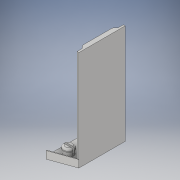
# Autodesk Inventor part: SOPORTE
Saved by Autodesk Inventor 2019 (Build 230136000, 136)
## iProperties
Created: 2020-12-03
Part Number: SOPORTE
Material: Generic
Document SubType Name: Modeling
Designer: mihai
Density: 1 g/cm^3
Appearance: Default
Author: mihai
Autodesk Inventor part; units mm, degrees
ref_plane "YZ Plane" through (0, 0, 0) normal (1, 0, 0) x (0, 1, 0)
ref_plane "XZ Plane" through (0, 0, 0) normal (0, 1, 0) x (-1, 0, 0)
ref_plane "XY Plane" through (0, 0, 0) normal (0, 0, 1) x (1, 0, 0)
sketch "Sketch1" plane through (0, 0, 0) normal (0, 1, 0) x (-1, 0, 0)
  line L0 (0, 0) -> (0, -30)
  circle A0 centre (0, 5) radius 5
  circle A1 centre (0, -35) radius 5
  line L1 (-5, 5) -> (-14, 5) construction
  line L2 (0, 10) -> (0, 15) construction
  line L3 (0, 10) -> (-14, 10) construction
  line L4 (5, 5) -> (10, 5) construction
  line L5 (-14, 5) -> (-11.1, 5) construction
  line L6 (0, 0) -> (-14, 0) construction
  line L7 (-11.1, 0) -> (-11.1, 1) construction
  line L8 (5, -35) -> (10, -35) construction
  line L9 (0, -40) -> (0, -45) construction
  line L10 (-5, -35) -> (-14, -35) construction
  line L11 (0, -40) -> (-14, -40) construction
  line L12 (0, -30) -> (-14, -30) construction
  line L13 (-11.1, -30) -> (-11.1, -31) construction
  line L14 (-14, 10) -> (0, 15)
  line L15 (0, 15) -> (10, 18.5714)
  line L16 (-14, -40) -> (0, -45)
  line L17 (0, -45) -> (10, -48.5714)
  line L18 (10, -48.5714) -> (10, 18.5714)
  line L19 (-14, 10) -> (-14, 5)
  line L20 (-11.1, 1) -> (-11.1, -31)
  line L21 (-14, -40) -> (-14, -35)
  line L22 (-14, 10) -> (-14, 3.9) construction
  line L23 (-14, -40) -> (-14, -33.9) construction
  line L24 (-11.1, 1) -> (-14, 4.45)
  line L25 (-11.1, -31) -> (-14, -34.45)
  line L26 (-14, 4.45) -> (-14, 5)
  line L27 (-14, -34.45) -> (-14, -35)
  dimension "d0" = 30
  dimension "d3" = 9
  dimension "d4" = 5
  dimension "d5" = 5
  dimension "d6" = 2.9
  dimension "d7" = 1
  dimension "d8" = 5
  dimension "d9" = 1
  dimension "d10" = 6.1
  dimension "d11" = 6.1
  constraints: 56 end point, 9 point on circle, 8 horizontal, 7 point on line, 5 vertical, 2 centre point, 2 collinear, 2 parallel, 2 tangent, 1 perpendicular
  measures "d0" distance of L0.start L0.end
  measures "d3" distance of L1.start L1.end
  measures "d4" distance of L2.start L2.end
  measures "d5" distance of L4.start L4.end
  measures "d6" distance of L1.end L5.end
  measures "d7" distance of L7.start L7.end
  measures "d8" distance of L9.start L9.end
  measures "d9" distance of L13.start L13.end
  measures "d10" distance of L3.end L22.end
  measures "d11" distance of L11.end L23.end
extrude "Extrusion3" add sketch "Sketch1" along normal blind 3
sketch "Sketch4" plane through (0, 3, 0) normal (0, 1, 0) x (1, 0, 0)
  circle A0 centre (0, 35) radius 5 projected
  circle A1 centre (0, -5) radius 5 projected
  point P0 (0, 0)
  constraints: 1 vertical alignment
sketch "Sketch5" plane through (0, 3, 0) normal (0, 1, 0) x (1, 0, 0)
  point P0 (0, 0)
extrude "Extrusion4" add sketch "Sketch4" along normal blind 5
sketch "Sketch6" plane through (0, 8, 5) normal (0, 1, 0) x (1, 0, 0)
  circle A0 centre (0, 0) radius 5.5
  circle A1 centre (0, 40) radius 5 projected
  circle A2 centre (0, 40) radius 5.5
  point P0 (0, 5)
  dimension "d20" = 11
  dimension "d21" = 11
  constraints: 2 centre point, 1 coincident
  measures "d20" diameter of A0
  measures "d21" diameter of A2
extrude "Extrusion5" add sketch "Sketch6" along normal blind 3 contours A0 | A1 | A2
fillet "Fillet1" radius 2 2 edges at (-5.5, 11, 5) (-5.5, 11, -35)
sketch "Sketch7" plane through (0, 11, 5) normal (0, 1, 0) x (1, 0, 0)
  circle A0 centre (0, 0) radius 3.5 projected
  circle A1 centre (0, 40) radius 3.5 projected
  circle A2 centre (0, 0) radius 5.5 projected
  line L0 (-5.5, 0) -> (-5.5, 1)
  line L1 (-5.5, 1) -> (5.5, 1)
  line L2 (5.5, 1) -> (5.5, -1)
  line L3 (5.5, -1) -> (-5.5, -1)
  line L4 (-5.5, -1) -> (-5.5, 0)
  line L5 (-5.5, 40) -> (-5.5, 41)
  line L6 (-5.5, 41) -> (5.5, 41)
  line L7 (5.5, 41) -> (5.5, 39)
  line L8 (5.5, 39) -> (-5.5, 39.0974)
  line L9 (-5.5, 39.0974) -> (-5.5, 40)
  circle A3 centre (0, 40) radius 5.5 projected
  point P0 (0, 5)
  dimension "d25" = 1
  dimension "d26" = 2
  dimension "d27" = 1
  dimension "d28" = 2
  constraints: 20 end point, 6 point on line, 5 perpendicular, 4 vertical, 2 horizontal alignment, 1 collinear, 1 other
  measures "d25" distance of L0.start L0.end
  measures "d26" distance of L1.end L2.end
  measures "d27" distance of L5.start L5.end
  measures "d28" distance of L6.end L7.end
extrude "Extrusion6" cut sketch "Sketch7" against normal blind 7 contours A0 L3 L1 | A0 L1 A2 L3 | A0 L3 A2 L1 | L1 L2 A2 | A2 L2 L3 | A2 L0 L1 | L3 L4 A2 | A1 L8 L6 | A1 L6 A3 L8 | A1 L8 A3 L6 | L6 L7 A3 | A3 L7 L8 | A3 L5 L6 | L8 L9 A3
fillet "Fillet2" radius 0.6 4 edges at (0, 4, 6) (0, 4, 4) (-0.0084, 4, -34.0488) (0, 4, -36)
sketch "Sketch8" plane through (0, 0, 0) normal (0, -1, 0) x (1, 0, 0)
  circle A0 centre (0, 5) radius 5 projected
  circle A1 centre (0, -35) radius 5 projected
  point P0 (0, 0)
  constraints: 1 vertical alignment
extrude "Extrusion7" add sketch "Sketch8" against normal blind 3
sketch "Sketch9" plane through (0, 3, 0) normal (0, 1, 0) x (1, 0, 0)
  circle A0 centre (0, 35) radius 5 projected
  circle A1 centre (0, -5) radius 5 projected
  line L0 (14, -10) -> (14, -4.45) projected
  line L1 (14, -4.45) -> (11.1, -1) projected
  line L2 (11.1, -1) -> (11.1, 31) projected
  line L3 (11.1, 31) -> (14, 34.45) projected
  line L4 (14, 34.45) -> (14, 40) projected
  line L5 (14, 40) -> (-10, 48.5714) projected
  line L6 (-10, 48.5714) -> (-10, -18.5714) projected
  line L7 (-10, -18.5714) -> (14, -10) projected
  line L8 (14, -10) -> (16, -10)
  line L9 (16, -10) -> (16, 40)
  line L10 (16, 40) -> (14, 40)
  point P0 (0, 0)
  dimension "d34" = 2
  constraints: 6 end point, 2 perpendicular, 1 horizontal
  measures "d34" distance of L0.start L8.end
extrude "Extrusion8" add sketch "Sketch9" along normal blind 105 contours L0 L1 L2 L3 L4 L10 L9 L8
sketch "Sketch10" plane through (0, 0, 0) normal (0, -1, 0) x (1, 0, 0)
  line L0 (14, 4.45) -> (14, 10) projected
  line L1 (14, 10) -> (-10, 18.5714) projected
  line L2 (-10, 18.5714) -> (-10, -48.5714) projected
  line L3 (-10, -48.5714) -> (14, -40) projected
  line L4 (14, -40) -> (14, -34.45) projected
  line L5 (14, -34.45) -> (11.1, -31) projected
  line L6 (11.1, -31) -> (11.1, 1) projected
  line L7 (11.1, 1) -> (14, 4.45) projected
  line L8 (14, 10) -> (16, 10) projected
  line L9 (14, 10) -> (14, 4.45) projected
  line L10 (14, 4.45) -> (11.1, 1) projected
  line L11 (11.1, 1) -> (11.1, -31) projected
  line L12 (11.1, -31) -> (14, -34.45) projected
  line L13 (14, -34.45) -> (14, -40) projected
  line L14 (16, -40) -> (14, -40) projected
  line L15 (16, 10) -> (16, -40) projected
  point P0 (0, 0)
extrude "Extrusion9" add sketch "Sketch10" against normal blind 3 contours L0 L8 L15 L14 L4 L5 L6 L7
fillet "Fillet3" radius 0.8 4 edges at (11.1, 55.5, 1) (14, 55.5, 4.45) (14, 55.5, -34.45) (11.1, 55.5, -31)
sketch "Sketch11" plane through (0, 3, 0) normal (0, 1, 0) x (1, 0, 0)
  arc A0 (13.8124, 34.2268) -> (14, 34.7416) centre (13.2, 34.7416) ccw projected
  line L0 (14, 34.7416) -> (14, 40) projected
  line L1 (14, 40) -> (-10, 48.5714) projected
  line L2 (-10, 48.5714) -> (-10, -18.5714) projected
  line L3 (-10, -18.5714) -> (14, -10) projected
  line L4 (14, -10) -> (14, -4.7416) projected
  arc A1 (14, -4.7416) -> (13.8124, -4.2268) centre (13.2, -4.7416) ccw projected
  line L5 (13.8124, -4.2268) -> (11.2876, -1.2232) projected
  arc A2 (11.1, -0.7084) -> (11.2876, -1.2232) centre (11.9, -0.7084) ccw projected
  line L6 (11.1, -0.7084) -> (11.1, 30.7084) projected
  arc A3 (11.2876, 31.2232) -> (11.1, 30.7084) centre (11.9, 30.7084) ccw projected
  line L7 (11.2876, 31.2232) -> (13.8124, 34.2268) projected
  circle A4 centre (0, -5) radius 5 projected
  circle A5 centre (0, 35) radius 5 projected
  line L8 (-10, 48.5714) -> (-10, -18.5714) projected
  line L9 (-10, 48.5714) -> (-10, 52.4265)
  line L10 (11.1, 40) -> (23.5531, 40)
  line L11 (16, 40) -> (14, 40) projected
  line L12 (16, 40) -> (-10, 49.2857)
  line L13 (14, -10) -> (19.1534, -10)
  line L14 (-10, -18.5714) -> (14, -10) projected
  line L15 (-10, -18.5714) -> (-10, -22.2627)
  line L16 (16, -10) -> (16, 40) projected
  line L17 (16, -10) -> (-10, -19.2857)
  point P0 (0, 0)
  constraints: 12 end point, 2 horizontal, 2 point on line, 2 vertical, 1 parallel
extrude "Extrusion10" add sketch "Sketch11" along normal blind 5 contours L1 L9 L12 L10 | L3 L13 L17 L15
sketch "Sketch12" plane through (0, 0, 0) normal (0, -1, 0) x (1, 0, 0)
  line L0 (14, -40) -> (16, -40) projected
  line L1 (14, -40) -> (-10, -48.5714) projected
  line L2 (-10, -49.2857) -> (-10, -48.5714) projected
  line L3 (16, -40) -> (-10, -49.2857) projected
  line L4 (-10, 18.5714) -> (-10, 19.2857) projected
  line L5 (-10, 18.5714) -> (14, 10) projected
  line L6 (16, 10) -> (14, 10) projected
  line L7 (-10, 19.2857) -> (16, 10) projected
  point P0 (0, 0)
extrude "Extrusion11" add sketch "Sketch12" against normal blind 3
body "Solid3"
